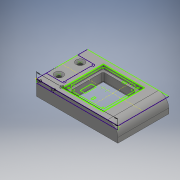
# Autodesk Inventor part: TNS_V3.1_Greiferbacke
Saved by Autodesk Inventor 2017 (Build 210142000, 142)
## iProperties
Created: 2015-08-26
Part Number: TNS_V3.1_Greiferbacke
Material: PVC, Unplasticized
Document SubType Name: Modeling
Designer: Sam
Density: 1.29 g/cm^3
Appearance: Smooth - White
Author: Sam
Autodesk Inventor part; units mm, degrees
ref_plane "YZ Plane" through (0, 0, 0) normal (1, 0, 0) x (0, 1, 0)
ref_plane "XZ Plane" through (0, 0, 0) normal (0, 1, 0) x (-1, 0, 0)
ref_plane "XY Plane" through (0, 0, 0) normal (0, 0, 1) x (1, 0, 0)
sketch "Unten" plane through (0, 0, 0) normal (0, 0, 1) x (1, 0, 0)
  line L0 (20.5633, 45) -> (20.5633, 5)
  line L1 (60.5633, 5) -> (60.5633, 45)
  line L2 (60.5633, 45) -> (20.5633, 45)
  line L3 (20.5633, 5) -> (60.5633, 5)
  line L4 (80, 50) -> (0, 50)
  line L5 (80, 0) -> (0, 0)
  line L6 (0, 40.5) -> (16, 40.5)
  line L7 (16, 37.5) -> (16, 12.5)
  line L8 (16, 9.5) -> (0, 9.5)
  line L9 (0, 9.5) -> (0, 40.5)
  line L10 (0, 50) -> (0, 0)
  line L11 (80, 50) -> (80, 0)
  circle A0 centre (23.5633, 8) radius 1
  circle A1 centre (57.5633, 42) radius 1
  line L12 (58.5633, 37.1716) -> (58.5633, 8.5)
  line L13 (57.0633, 7) -> (28.3918, 7)
  line L14 (22.5633, 12.8284) -> (22.5633, 41.5)
  line L15 (24.0633, 43) -> (52.7349, 43)
  line L16 (20.0633, 45.5) -> (61.0633, 45.5)
  line L17 (61.0633, 4.5) -> (20.0633, 4.5)
  arc A2 (57.0633, 7) -> (58.5633, 8.5) centre (57.0633, 8.5) ccw
  arc A3 (24.0633, 43) -> (22.5633, 41.5) centre (24.0633, 41.5) ccw
  line L18 (23.1491, 11.4142) -> (26.9776, 7.5858)
  line L19 (54.1491, 42.4142) -> (57.9776, 38.5858)
  arc A4 (16, 37.5) -> (16, 40.5) centre (16, 39) ccw
  arc A5 (16, 9.5) -> (16, 12.5) centre (16, 11) ccw
  line L20 (20.0633, 45.5) -> (20.0633, 4.5)
  line L21 (61.0633, 4.5) -> (61.0633, 45.5)
  line L22 (0, 25) -> (80, 25) construction
  arc A6 (22.5633, 12.8284) -> (23.1491, 11.4142) centre (24.5633, 12.8284) ccw
  arc A7 (26.9776, 7.5858) -> (28.3918, 7) centre (28.3918, 9) ccw
  arc A8 (58.5633, 37.1716) -> (57.9776, 38.5858) centre (56.5633, 37.1716) ccw
  arc A9 (54.1491, 42.4142) -> (52.7349, 43) centre (52.7349, 41) ccw
  line L23 (50, 0) -> (50, 50) construction
  line L24 (48, 39) -> (48, 40.8)
  line L25 (48, 40.8) -> (44.6, 40.8)
  line L26 (44.6, 40.8) -> (44.6, 39)
  line L27 (44.6, 39) -> (48, 39)
  line L28 (36.2594, 22.5) -> (31.2594, 22.5)
  line L29 (31.2594, 22.5) -> (31.2594, 11.5)
  line L30 (31.2594, 11.5) -> (36.2594, 11.5)
  line L31 (36.2594, 11.5) -> (36.2594, 22.5)
  line L32 (43.6, 9.7) -> (43.6, 13.1)
  line L33 (43.6, 13.1) -> (45.4, 13.1)
  line L34 (45.4, 13.1) -> (45.4, 9.7)
  line L35 (45.4, 9.7) -> (43.6, 9.7)
  point P0 (0, 0)
  point P1 (7.5, 14.5)
  point P2 (7.5, 35.5)
  point P3 (58.5633, 38)
  point P4 (27.5633, 7)
  point P5 (53.5633, 43)
  point P6 (22.5633, 12)
  point P7 (40.5633, 25)
  point P8 (44.7594, 25)
  dimension "d0" = 40
  dimension "d1" = 40
  dimension "d185" = 80
  dimension "d196" = 21
  dimension "d217" = 31
  dimension "d267" = 14.5
  dimension "d268" = 14.5
  dimension "d269" = 50
  dimension "d308" = 9.5
  dimension "d329" = 3
  dimension "d341" = 3
  dimension "d342" = 3
  dimension "d343" = 2
  dimension "d344" = 2
  dimension "d390" = 3
  dimension "d391" = 3
  dimension "d419" = 2
  dimension "d420" = 2
  dimension "d421" = 2
  dimension "d423" = 1.5
  dimension "d424" = 1.5
  dimension "d427" = 0.5
  dimension "d428" = 0.5
  dimension "d431" = 3.5
  dimension "d432" = 3.5
  dimension "d450" = 3.5
  dimension "d451" = 3.5
  dimension "d463" = 3
  dimension "d464" = 1.5
  dimension "d465" = 3
  dimension "d466" = 1.5
  dimension "d482" = 2
  dimension "d515" = 5
  dimension "d516" = 11
  dimension "d517" = 3.4
  dimension "d518" = 1.8
  dimension "d519" = 3.4
  dimension "d520" = 1.8
  dimension "d521" = 7.5
  dimension "d522" = 16
  constraints: 72 end point, 16 point on circle, 13 point on line, 10 centre point, 10 parallel, 8 tangent, 5 perpendicular, 3 equal radius, 3 horizontal, 3 vertical, 2 coincident, 2 midpoint
  measures "d0" distance of L2.start L1.start
  measures "d1" distance of L0.end L1.start
  measures "d185" distance of L5.start L5.end
  measures "d196" distance of point (7.5, 35.5) point (7.5, 14.5)
  measures "d217" distance of L6.end L8.start
  measures "d267" distance from line of L4 point (7.5, 35.5)
  measures "d268" distance from line of L5 point (7.5, 14.5)
  measures "d269" distance of L4.end L5.end
  measures "d308" distance between parallel lines of L5 L8
  measures "d329" distance from line of L2 point (57.563, 42)
  measures "d341" distance from line of L1 point (57.563, 42)
  measures "d342" distance from line of L0 point (23.563, 8)
  measures "d343" diameter of A0
  measures "d344" diameter of A1
  measures "d390" distance from line of L3 A0.centre
  measures "d391" distance from line of L2 A1.centre
  measures "d419" distance between parallel lines of L0 L14
  measures "d420" distance between parallel lines of L1 L12
  measures "d421" distance between parallel lines of L2 L15
  measures "d423" radius of A3
  measures "d424" radius of A2
  measures "d427" distance between parallel lines of L2 L16
  measures "d428" distance between parallel lines of L17 L3
  measures "d431" distance from line of L1 A2.centre
  measures "d432" distance from line of L3 A2.centre
  measures "d450" distance from line of L0 A3.centre
  measures "d451" distance from line of L2 A3.centre
  measures "d463" diameter of A4
  measures "d464" distance from line of L6 A4.centre
  measures "d465" diameter of A5
  measures "d466" distance from line of L8 A5.centre
  measures "d482" radius of A6
  measures "d515" distance of L31.start L30.start
  measures "d516" distance of L30.start L29.start
  measures "d517" distance of L26.end L27.end
  measures "d518" distance of L26.start L26.end
  measures "d519" distance of L33.end L34.end
  measures "d520" distance of L33.start L33.end
  measures "d521" distance from line of L10 point (7.5, 35.5)
  measures "d522" distance between parallel lines of L10 L7
extrude "Extrusion40" add sketch "Unten" against normal blind 15 contours L11 L5 L10 L8 A5 L7 A4 L6 L4 | L16 L21 L17 L20
extrude "Extrusion46" add sketch "Unten" against normal blind 12 contours L2 L1 L3 L0
extrude "Extrusion48" cut sketch "Unten" against normal blind 4.4 contours L2 L1 L3 L0 | L12 A2 L13 A7 L18 A6 L14 A3 L15 A9 L19 A8 | L16 L21 L17 L20 | L27 L26 L25 L24 | L31 L30 L29 L28 | L32 L33 L34 L35
extrude "Extrusion41" add sketch "Unten" against normal blind 6 contours L6 A4 L7 A5 L8 L9
hole "Hole14" at (7.5, 14.5, 0) at (7.5, 35.5, 0) direction (0, 0, -1) diameter 4 end through all
chamfer "Chamfer8" distance 2 angle 45 2 edges at (7.5, 37.5, 0) (7.5, 16.5, 0)
sketch "Side" plane through (0, 0, 0) normal (0, -1, 0) x (1, 0, 0)
  line L0 (80, 0) -> (0, 0)
  line L1 (0, -3.6) -> (80, -3.6)
  line L2 (80, -3.6) -> (80, 0)
  line L3 (0, -3.6) -> (0, 0)
  point P0 (0, 0)
  dimension "d412" = 3.6
  dimension "d443" = 80
  dimension "d479" = 80
  constraints: 8 end point, 1 horizontal, 1 parallel
  measures "d412" distance between parallel lines of L0 L1
  measures "d443" distance of L0.start L0.end
  measures "d479" distance of L1.start L1.end
fillet "Fillet4" radius 10 1 edges at (80, 25, 0)
body "Solid5"
